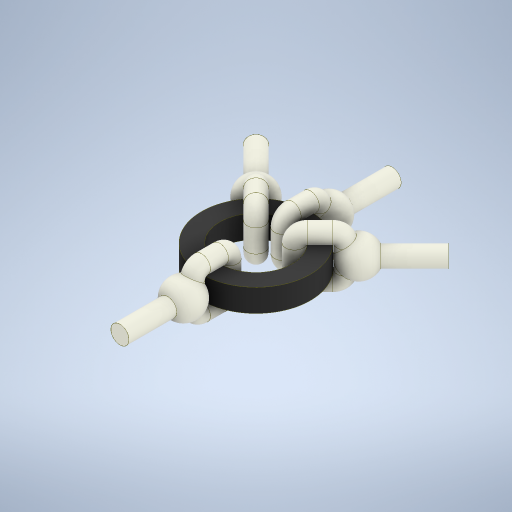
# Autodesk Inventor part: dummy_expansion_ring_4.8mm_w_string
Saved by Autodesk Inventor 2024.3 (Build 283343000, 343)
## iProperties
Created: 2024-06-24
Part Number: dummy_expansion_ring_4.8mm_w_string
Material: 일반
Document SubType Name: Modeling
Designer: Gihyeok Na
Density: 1 g/cm^3
Appearance: Smooth - Ivory
Author: Gihyeok Na
Autodesk Inventor part; units mm, degrees
ref_plane "YZ Plane" through (0, 0, 0) normal (1, 0, 0) x (0, 1, 0)
ref_plane "XZ Plane" through (0, 0, 0) normal (0, 1, 0) x (-1, 0, 0)
sketch "스케치1" plane through (0, 0, 0) normal (0, 1, 0) x (-1, 0, 0)
  circle A0 centre (0, 0) radius 1.6
  circle A1 centre (0, 0) radius 2.4
  dimension "d0" = 3.2
  dimension "d1" = 4.8
  constraints: 2 centre point, 2 coincident
  measures "d0" diameter of A0
  measures "d1" diameter of A1
extrude "돌출1" add sketch "스케치1" along normal blind 1
sketch "Sketch2" plane through (0, 0, 0) normal (1, 0, 0) x (0, 1, 0)
  line L0 (0, 1.2) -> (1, 1.2)
  line L1 (1.4, 1.6) -> (1.4, 2.4)
  line L2 (1, 2.8) -> (0, 2.8)
  line L3 (-0.4, 2.4) -> (-0.4, 1.6)
  line L4 (0, 2.4) -> (1, 2.4) projected
  line L5 (0, -2.4) -> (0, 2.4) projected
  line L6 (1, -2.4) -> (1, 2.4) projected
  line L7 (2.0485, 0) -> (-0.9221, 0) construction
  line L8 (1, 1.6) -> (0, 1.6) projected
  arc A0 (1.4, 2.4) -> (1, 2.8) centre (1, 2.4) ccw
  arc A1 (0, 2.8) -> (-0.4, 2.4) centre (0, 2.4) ccw
  arc A2 (-0.4, 1.6) -> (0, 1.2) centre (0, 1.6) ccw
  arc A3 (1, 1.2) -> (1.4, 1.6) centre (1, 1.6) ccw
  line L9 (0, -1.2) -> (1, -1.2)
  line L10 (1.4, -1.6) -> (1.4, -2.4)
  line L11 (1, -2.8) -> (0, -2.8)
  line L12 (-0.4, -2.4) -> (-0.4, -1.6)
  line L13 (0, -2.4) -> (1, -2.4)
  line L14 (1, -1.6) -> (0, -1.6)
  arc A4 (1, -2.8) -> (1.4, -2.4) centre (1, -2.4) ccw
  arc A5 (-0.4, -2.4) -> (0, -2.8) centre (0, -2.4) ccw
  arc A6 (0, -1.2) -> (-0.4, -1.6) centre (0, -1.6) ccw
  arc A7 (1.4, -1.6) -> (1, -1.2) centre (1, -1.6) ccw
  circle A8 centre (0.5, -3.2) radius 0.8
  circle A9 centre (0.5, 3.2) radius 0.8
  line L15 (1.3, -3.2) -> (-0.3, -3.2)
  line L16 (-0.3, 3.2) -> (1.3, 3.2)
  point P0 (0, 0)
  point P1 (0.5, 2.4)
  point P2 (0.5, -2.4)
  dimension "d4" = 0.5
  dimension "d8" = 0.4
  dimension "d9" = 0.4
  dimension "d10" = 0.4
  dimension "d20" = 1.6
  dimension "d21" = 0.8
  dimension "d22" = 1.6
  dimension "d23" = 0.8
  constraints: 26 end point, 20 point on circle, 15 symmetric about line, 10 centre point, 8 coincident, 5 point on line, 3 horizontal, 3 parallel, 2 midpoint, 1 perpendicular, 1 tangent, 4 other
  measures "d4" distance from line of L5 point (0.5, 2.4)
  measures "d8" distance between parallel lines of L6 L1
  measures "d9" distance between parallel lines of L5 L3
  measures "d10" distance between parallel lines of L4 L2
  measures "d20" diameter of A8
  measures "d21" distance from line of L13 A8.centre
  measures "d22" diameter of A9
  measures "d23" distance from line of A9.centre L4
sketch "Sketch3" plane through (0, 0, 0) normal (0, 1, 0) x (-1, 0, 0)
  line L0 (0, 2.8) -> (0, 2.4) projected
  circle A0 centre (0, 2.8) radius 0.39
  line L1 (0, -2.4) -> (0, -2.8) projected
  circle A1 centre (0, -2.8) radius 0.39
  point P0 (0, 0)
  dimension "d12" = 0.78
  dimension "d15" = 0.78
  constraints: 2 centre point, 2 coincident
  measures "d12" diameter of A0
  measures "d15" diameter of A1
sweep "Sweep1" add profiles "Sketch3" path "Sketch2" path curves L2 A0 L1 A3 L0 A2 L3 A1 contours A0
sweep "Sweep2" add profiles "Sketch3" path "Sketch2" path curves L11 A4 L10 A7 L9 A6 L12 A5 contours A1
revolve "Revolution1" add sketch "Sketch2" angle 360 about axis through (0, 1.3, -3.2) along (0, -1, 0) contours L15 A8
revolve "Revolution2" add sketch "Sketch2" angle 360 about axis through (0, -0.3, 3.2) along (0, 1, 0) contours A9 L16
ref_plane "Work Plane2" through (0, 0.5, -4) normal (0, 0, 1) x (1, 0, 0)
ref_plane "Work Plane1" through (0, 0.5, 4) normal (0, 0, 1) x (1, 0, 0)
sketch "Sketch5" plane through (0, 0.5, 4) normal (0, 0, 1) x (1, 0, 0)
  circle A0 centre (0, 0) radius 0.4
  point P0 (0, -0.5)
  point P1 (0.3776, -0.5)
  point P2 (-0.3776, -0.5)
  point P3 (-0.3776, 0.5)
  point P4 (0.3776, 0.5)
  dimension "d27" = 0.8
  constraints: 4 horizontal alignment, 1 centre point, 1 coincident
  measures "d27" diameter of A0
extrude "Extrusion2" add sketch "Sketch5" along normal blind 2 and the other way blind 1
sketch "Sketch6" plane through (0, 0.5, -4) normal (0, 0, 1) x (1, 0, 0)
  circle A0 centre (0, 0) radius 0.4
  point P0 (0, -0.5)
  dimension "d32" = 0.8
  constraints: 1 centre point
  measures "d32" diameter of A0
extrude "Extrusion3" add sketch "Sketch6" along normal blind 0.5 and the other way blind 2
pattern_circular "Circular Pattern1" count 2 over 45 about axis through (0, 0, 0) along (0, 1, 0) of "Sweep2", "Extrusion3", "Revolution1"
pattern_circular "Circular Pattern2" count 2 over 45 about axis through (0, 0, 0) along (0, -1, 0) of "Sweep2", "Revolution1", "Extrusion3"
